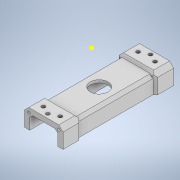
# Autodesk Inventor part: magnet handle top
Saved by Autodesk Inventor 2022 (Build 260153000, 153)
## iProperties
Created: 2022-12-16
Part Number: magnet handle top
Material: Generic
Document SubType Name: Modeling
Designer: chris
Density: 1 g/cm^3
Appearance: Default
Author: chris
Autodesk Inventor part; units mm, degrees
ref_plane "YZ Plane" through (0, 0, 0) normal (1, 0, 0) x (0, 1, 0)
ref_plane "XZ Plane" through (0, 0, 0) normal (0, 1, 0) x (-1, 0, 0)
ref_plane "XY Plane" through (0, 0, 0) normal (0, 0, 1) x (1, 0, 0)
sketch "Sketch1" plane through (0, 0, 0) normal (0, 0, 1) x (1, 0, 0)
  line L0 (0, 0) -> (80, 0)
  line L1 (80, 0) -> (80, 125.359)
  line L2 (60, 200) -> (80, 125.359)
  line L3 (60, 200) -> (137.2741, 200) construction
  line L4 (0, 0) -> (0, 125.359)
  line L5 (20, 200) -> (0, 125.359)
  line L6 (84, 125.8856) -> (84, -4)
  line L7 (84, -4) -> (-4, -4)
  line L8 (-4, -4) -> (-4, 125.8856)
  line L9 (-4, 125.8856) -> (16.9307, 204)
  line L10 (63.0693, 204) -> (84, 125.8856)
  line L11 (20, 204) -> (20, 200)
  line L12 (60, 200) -> (60, 204)
  line L13 (16.9307, 204) -> (20, 204)
  line L14 (60, 204) -> (63.0693, 204)
  point P0 (40, 0)
  dimension "d0" = 80
  dimension "d4" = 75
  dimension "d5" = 4
  constraints: 30 end point, 4 perpendicular, 2 horizontal, 1 equal length, 1 midpoint, 1 vertical, 3 other
  measures "d0" distance of L0.start L0.end
  measures "d4" angle of L2 L3
  measures "d5" distance between parallel lines of L2 L10
extrude "Extrusion1" add sketch "Sketch1" along normal blind 70
sketch "Sketch2" plane through (0, 0, 0) normal (0, 0, -1) x (-1, 0, 0)
  line L0 (-16.9307, 204) -> (4, 125.8856) projected
  line L1 (-84, 125.8856) -> (-63.0693, 204) projected
  line L2 (-16.9307, 204) -> (-63.0693, 204)
  line L3 (-80, 125.359) -> (-80, 0) projected
  line L4 (-60, 200) -> (-80, 125.359) projected
  line L5 (-60, 204) -> (-60, 200) projected
  line L6 (-63.0693, 204) -> (-60, 204) projected
  line L7 (-84, 125.8856) -> (-63.0693, 204) projected
  line L8 (-84, -4) -> (-84, 125.8856) projected
  line L9 (4, -4) -> (-84, -4) projected
  line L10 (4, 125.8856) -> (4, -4) projected
  line L11 (-16.9307, 204) -> (4, 125.8856) projected
  line L12 (-20, 204) -> (-16.9307, 204) projected
  line L13 (-20, 200) -> (-20, 204) projected
  line L14 (0, 125.359) -> (-20, 200) projected
  line L15 (0, 0) -> (0, 125.359) projected
  line L16 (-80, 0) -> (0, 0) projected
  constraints: 2 end point, 1 horizontal
extrude "Extrusion2" add sketch "Sketch2" along normal blind 3
chamfer "Chamfer1" distance 5 angle 45 5 edges at (40, -4, -3) (84, 60.9428, -3) (-4, 60.9428, -3) (6.4653, 164.9428, -3) (73.5347, 164.9428, -3)
chamfer "Chamfer2" distance 3 angle 45 7 edges at (20, 202, 0) (10, 162.6795, 0) (60, 202, 0) (70, 162.6795, 0) (80, 62.6795, 0) (0, 62.6795, 0) (40, 0, 0)
chamfer "Chamfer3" distance 3 angle 45 4 edges at (84, -4, 36) (-4, -4, 36) (0, 0, 36.5) (80, 0, 36.5)
sketch "Sketch3" plane through (0, 0, 70) normal (0, 0, 1) x (1, 0, 0)
  line L0 (77, 0) -> (78.5, 1.5) projected
  line L1 (81, -4) -> (82.5, -2.5) projected
  line L2 (78.5, 1.5) -> (82.5, -2.5)
  line L3 (79, 1) -> (82.5, -2.5) projected
  circle A0 centre (80.75, -0.75) radius 1
  line L4 (-4, -1) -> (-2.5, -2.5) projected
  line L5 (-2.5, -2.5) -> (1.5, 1.5)
  line L6 (0, 3) -> (3, 0) projected
  line L7 (1, 1) -> (-2.5, -2.5) projected
  circle A1 centre (-0.75, -0.75) radius 1
  line L8 (3, 124.964) -> (0, 125.359) projected
  line L9 (16.9307, 204) -> (-4, 125.8856) projected
  line L10 (80, 125.359) -> (77, 124.964) projected
  line L11 (84, -1) -> (84, 125.8856) projected
  line L12 (1, 125.2273) -> (-4, 125.8856) projected
  circle A2 centre (82, 125.6223) radius 1
  circle A3 centre (-2, 125.6223) radius 1
  point P0 (0, 0)
  dimension "d19" = 2
  dimension "d20" = 2
  dimension "d22" = 2
  dimension "d23" = 2
  constraints: 4 centre point, 4 end point, 3 midpoint, 1 perpendicular, 1 point on line
  measures "d19" diameter of A0
  measures "d20" diameter of A1
  measures "d22" diameter of A2
  measures "d23" diameter of A3
extrude "Extrusion3" cut sketch "Sketch3" against normal blind 5
sketch "Sketch4" plane through (22.1071, 204, -3) normal (0, 1, 0) x (1, 0, 0)
  line L0 (35.7859, 0) -> (40.9622, -5) projected
  line L1 (38.374, -2.5) -> (36.3929, -4.5)
  line L2 (34.8929, -3) -> (37.8929, -6) projected
  circle A0 centre (37.3835, -3.5) radius 1
  line L3 (-21.1071, 0) -> (56.8929, 0) projected
  line L4 (17.8929, 0) -> (17.8929, -26)
  circle A1 centre (-1.5976, -3.5) radius 1
  point P0 (-22.1071, -3)
  dimension "d26" = 2
  constraints: 4 end point, 4 midpoint, 2 centre point, 1 symmetric about line, 1 vertical, 1 other
  measures "d26" diameter of A0
extrude "Extrusion4" cut sketch "Sketch4" against normal blind 15
sketch "Sketch5" plane through (0, 0, 0) normal (0, 0, 1) x (1, 0, 0)
  line L0 (77, 3) -> (3, 3) projected
  line L1 (40, 3) -> (40, 43)
  line L2 (40, 43) -> (40, 113)
  line L3 (40, 78) -> (20, 78)
  line L4 (20, 78) -> (20, 55.5)
  line L5 (20, 55.5) -> (60, 55.5)
  line L6 (60, 55.5) -> (60, 100.5)
  line L7 (60, 100.5) -> (20, 100.5)
  line L8 (20, 100.5) -> (20, 78)
  line L9 (40, 78) -> (70, 78)
  line L10 (70, 78) -> (70, 98)
  circle A0 centre (70, 98) radius 1
  line L11 (70, 78) -> (70, 58)
  circle A1 centre (70, 58) radius 1
  circle A2 centre (10, 98) radius 1
  circle A3 centre (10, 58) radius 1
  line L12 (40, 113) -> (40, 133)
  line L13 (40, 133) -> (63.1521, 133)
  line L14 (63.1521, 133) -> (63.1521, 155.7076)
  circle A4 centre (63.1521, 155.7076) radius 1.5
  circle A5 centre (63.1521, 133) radius 1.5
  circle A6 centre (16.8479, 155.7076) radius 1.5
  circle A7 centre (16.8479, 133) radius 1.5
  point P0 (0, 0)
  dimension "d29" = 40
  dimension "d30" = 70
  dimension "d31" = 20
  dimension "d32" = 22.5
  dimension "d33" = 40
  dimension "d34" = 45
  dimension "d35" = 30
  dimension "d36" = 20
  dimension "d37" = 2
  dimension "d38" = 20
  dimension "d39" = 2
  dimension "d40" = 20
  dimension "d41" = 23.1521
  dimension "d42" = 22.7076
  dimension "d43" = 3
  dimension "d44" = 3
  constraints: 28 end point, 8 centre point, 5 perpendicular, 5 vertical, 4 coincident, 4 symmetric about line, 3 horizontal, 2 midpoint, 1 point on line, 4 other
  measures "d29" distance of L1.start L1.end
  measures "d30" distance of L1.end L2.end
  measures "d31" distance of L3.start L3.end
  measures "d32" distance of L3.end L4.end
  measures "d33" distance of L4.end L5.end
  measures "d34" distance of L5.end L6.end
  measures "d35" distance of L3.start L9.end
  measures "d36" distance of L9.end L10.end
  measures "d37" diameter of A0
  measures "d38" distance of L9.end L11.end
  measures "d39" diameter of A1
  measures "d40" distance of L2.end L12.end
  measures "d41" distance of L12.end L13.end
  measures "d42" distance of L13.end L14.end
  measures "d43" diameter of A4
  measures "d44" diameter of A5
extrude "Extrusion5" cut sketch "Sketch5" against normal blind 40
sketch "Sketch7" plane through (-1, -4, 2) normal (0, -1, 0) x (1, 0, 0)
  line L0 (78, 68) -> (4, 68) projected
  line L1 (41, 68) -> (41, 34)
  line L2 (54.7, 34) -> (27.3, 34)
  line L3 (54.7, 34) -> (54.7, 20.8)
  line L4 (54.7, 20.8) -> (27.3, 20.8)
  line L5 (27.3, 34) -> (27.3, 20.8)
  point P0 (1, -2)
  dimension "d47" = 27.4
  dimension "d48" = 34
  dimension "d49" = 13.2
  constraints: 10 end point, 3 vertical, 2 midpoint, 1 coincident, 1 horizontal, 1 horizontal alignment
  measures "d47" distance of L2.start L2.end
  measures "d48" distance of L1.start L1.end
  measures "d49" distance of L2.start L3.end
extrude "Extrusion6" cut sketch "Sketch7" against normal blind 27.4
sketch "Sketch8" plane through (-4, 125.8856, 2) normal (-0.9659258, 0.258819, 0) x (0, 0, 1)
  line L0 (-2, 13.7678) -> (-2, 10.7678) projected
  line L1 (-2, 35.7017) -> (-2, 32.7017) projected
  line L2 (3.9828, 34.5121) -> (3.9828, 12.5782)
  line L3 (3.9828, 23.5451) -> (5.9828, 23.5451)
  line L4 (5.9828, 23.5451) -> (12.9828, 23.5451)
  line L5 (12.9828, 23.5451) -> (12.9828, 30.2951)
  line L6 (12.9828, 30.2951) -> (12.9828, 16.7951)
  line L7 (12.9828, 16.7951) -> (5.9828, 16.7951)
  line L8 (5.9828, 16.7951) -> (5.9828, 29.9848)
  line L9 (5.9828, 29.9848) -> (12.9828, 30.2951)
  point P0 (-2, -120.5609)
  point P1 (12.9828, 30.2951)
  dimension "d52" = 2
  dimension "d53" = 7
  dimension "d54" = 6.75
  dimension "d55" = 13.5
  constraints: 16 end point, 3 perpendicular, 3 point on line, 1 coincident, 1 horizontal, 1 midpoint, 1 vertical
  measures "d52" distance of L3.start L3.end
  measures "d53" distance of L3.end L4.end
  measures "d54" distance of L4.end L5.end
  measures "d55" distance of L5.end L6.end
extrude "Extrusion7" cut sketch "Sketch8" against normal blind 9
chamfer "Chamfer4" distance 1 angle 45 4 edges at (5.7728, 154.6308, 14.9828) (2.2788, 141.5908, 14.9828) (2.2788, 141.5908, 7.9828) (5.6925, 154.331, 7.9828)
sketch "Sketch9" plane through (-4, 125.8856, 2) normal (-1, 0, 0) x (0, 0, 1)
  line L0 (1, -0.5266) -> (1, -122.8856) projected
  line L1 (1, -48.8247) -> (7.6436, -48.8247)
  line L2 (7.6436, -48.8247) -> (7.6436, -34.3247)
  line L3 (7.6436, -34.3247) -> (7.6436, -63.3247)
  circle A0 centre (7.6436, -34.3247) radius 2
  circle A1 centre (7.6436, -63.3247) radius 2
  point P0 (-2, -125.8856)
  dimension "d61" = 14.5
  dimension "d62" = 29
  dimension "d63" = 4
  dimension "d64" = 4
  constraints: 6 end point, 2 centre point, 2 coincident, 2 point on line, 1 horizontal, 1 perpendicular
  measures "d61" distance of L1.end L2.end
  measures "d62" distance of L2.end L3.end
  measures "d63" diameter of A0
  measures "d64" diameter of A1
extrude "Extrusion8" cut sketch "Sketch9" against normal blind 999
sketch "Sketch17" plane through (0, 0, -3) normal (0, 0, -1) x (-1, 0, 0)
  line L0 (-60, 55.5) -> (-60, 100.5) projected
  line L1 (-60, 78) -> (-77, 78)
  line L2 (-77, 124.964) -> (-77, 3) projected
  line L3 (-77, 78) -> (-77, 43)
  line L4 (-77, 78) -> (-77, 113)
  line L5 (-60, 55.5) -> (-20, 55.5) projected
  line L6 (-40, 55.5) -> (-40, 37.7198)
  line L7 (-20, 55.5) -> (-20, 100.5)
  line L8 (-20, 78) -> (-3, 78)
  line L9 (-3, 78) -> (-3, 43)
  line L10 (-3, 78) -> (-3, 113)
  line L11 (-20, 55.5) -> (-60, 55.5)
  line L12 (-77, 43) -> (-3, 43)
  line L13 (-3, 3) -> (-3, 124.964) projected
  line L14 (-3, 113) -> (-77, 113)
  line L15 (-79, 1) -> (-79, 125.2273) projected
  circle A0 centre (-63.1521, 133) radius 1.5 projected
  circle A1 centre (-70, 98) radius 1 projected
  circle A2 centre (-10, 58) radius 1 projected
  circle A3 centre (-16.8479, 133) radius 1.5 projected
  circle A4 centre (-63.1521, 155.7076) radius 1.5 projected
  circle A5 centre (-70, 58) radius 1 projected
  circle A6 centre (-10, 98) radius 1 projected
  circle A7 centre (-16.8479, 155.7076) radius 1.5 projected
  line L16 (-20, 55.5) -> (-60, 55.5) projected
  line L17 (-60, 55.5) -> (-60, 100.5) projected
  line L18 (-60, 100.5) -> (-20, 100.5) projected
  line L19 (-20, 100.5) -> (-20, 55.5) projected
  line L20 (-79, 125.2273) -> (-57.8929, 204) projected
  line L21 (-79, 1) -> (-79, 125.2273) projected
  line L22 (-1, 1) -> (-79, 1) projected
  line L23 (-1, 125.2273) -> (-1, 1) projected
  line L24 (-22.1071, 204) -> (-1, 125.2273) projected
  line L25 (-22.1071, 204) -> (-57.8929, 204) projected
  point P0 (0, 0)
  dimension "d106" = 35
  dimension "d107" = 35
  constraints: 22 end point, 7 symmetric about line, 3 perpendicular, 3 vertical, 2 midpoint, 1 point on line
  measures "d106" distance of L1.end L3.end
  measures "d107" distance of L1.end L4.end
extrude "Extrusion16" add sketch "Sketch17" along normal blind 3 contours L5 L6 L12 L2 L1 L0 | L0 L18 L7 L5 | L1 L2 L14 L10 L8 L7 L18 L0 | L5 L7 L8 L9 L12 L6
sketch "Sketch18" plane through (0, 0, 70) normal (0, 0, 1) x (1, 0, 0)
  line L0 (-145.0841, -156.9657) -> (0, 339.906)
  line L1 (0, 339.906) -> (209.9789, 212.1699)
  line L2 (209.9789, 212.1699) -> (104.9894, -207.8436)
  line L3 (104.9894, -207.8436) -> (-145.0841, -156.9657)
  point P0 (0, 0)
  constraints: 8 end point
extrude "Extrusion17" cut sketch "Sketch18" against normal blind 73
sketch "Sketch19" plane through (0, 0, -3) normal (0, 0, 1) x (1, 0, 0)
  line L0 (3, 113) -> (77, 113) projected
  line L1 (77, 43) -> (3, 43) projected
  line L2 (40, 43) -> (40, 113)
  line L3 (40, 78) -> (25, 78)
  line L4 (25, 78) -> (25, 63)
  line L5 (25, 63) -> (40, 63)
  line L6 (40, 63) -> (55, 63)
  line L7 (55, 63) -> (55, 93)
  line L8 (55, 93) -> (25, 93)
  line L9 (25, 93) -> (25, 78)
  line L10 (22, 78) -> (22, 60)
  line L11 (22, 60) -> (40, 60)
  line L12 (40, 60) -> (58, 60)
  line L13 (58, 60) -> (58, 96)
  line L14 (58, 96) -> (22, 96)
  line L15 (22, 96) -> (22, 78)
  point P0 (0, 0)
  dimension "d112" = 15
  dimension "d113" = 15
  dimension "d114" = 15
  dimension "d115" = 15
  dimension "d116" = 30
  dimension "d117" = 3
  constraints: 28 end point, 6 perpendicular, 3 midpoint, 3 point on line, 1 horizontal, 5 other
  measures "d112" distance of L3.start L3.end
  measures "d113" distance of L3.end L4.end
  measures "d114" distance of L4.end L5.end
  measures "d115" distance of L5.end L6.end
  measures "d116" distance of L6.end L7.end
  measures "d117" distance between parallel lines of L9 L15
extrude "Extrusion18" add sketch "Sketch19" along normal blind 73 contours L11 L10 L15 L14 L2 L8 L9 L4 L5 | L2 L6 L7 L8 L14 L13 L12
sketch "Sketch20" plane through (0, 0, -3) normal (0, 0, 1) x (1, 0, 0)
  line L0 (25, 93) -> (25, 63) projected
  line L1 (25, 63) -> (55, 63) projected
  line L2 (55, 63) -> (55, 93) projected
  line L3 (55, 93) -> (25, 93) projected
  point P0 (0, 0)
extrude "Extrusion19" cut sketch "Sketch20" against normal blind 73
chamfer "Chamfer7" distance 3 angle 45 8 edges at (58, 60, 33.5) (25, 93, 32) (58, 96, 33.5) (55, 63, 32) (22, 96, 33.5) (55, 93, 32) (25, 63, 32) (22, 60, 33.5)
chamfer "Chamfer8" distance 3 angle 45 4 edges at (3, 78, -3) (40, 43, -3) (77, 78, -3) (40, 113, -3)
sketch "Sketch21" plane through (25, 96, -3) normal (0, 1, 0) x (1, 0, 0)
  line L0 (0, -73) -> (0, 0) projected
  line L1 (30, -73) -> (0, -73) projected
  line L2 (30, 0) -> (30, -73) projected
  line L3 (0, 0) -> (30, 0) projected
  line L4 (0, -73) -> (0, 3) projected
  line L5 (0, -35) -> (30, -35)
  line L6 (30, -73) -> (30, 0) projected
  circle A0 centre (15, -35) radius 9.425
  point P0 (-25, -3)
  dimension "d128" = 18.85
  constraints: 2 end point, 2 midpoint, 1 centre point, 1 perpendicular, 1 point on line
  measures "d128" diameter of A0
extrude "Extrusion20" cut sketch "Sketch21" against normal blind 3 contours A0 L5 | L5 A0
sketch "Sketch22" plane through (0, 0, 70) normal (0, 0, 1) x (1, 0, 0)
  line L0 (25, 60) -> (22, 63) projected
  line L1 (25, 60) -> (55, 60) projected
  line L2 (58, 63) -> (55, 60) projected
  line L3 (58, 63) -> (58, 93) projected
  line L4 (55, 96) -> (58, 93) projected
  line L5 (55, 96) -> (25, 96) projected
  line L6 (22, 93) -> (25, 96) projected
  line L7 (22, 93) -> (22, 63) projected
  line L8 (28, 93) -> (52, 93) projected
  line L9 (55, 90) -> (52, 93) projected
  line L10 (55, 90) -> (55, 66) projected
  line L11 (52, 63) -> (55, 66) projected
  line L12 (52, 63) -> (28, 63) projected
  line L13 (25, 66) -> (28, 63) projected
  line L14 (25, 66) -> (25, 90) projected
  line L15 (28, 93) -> (25, 90) projected
  line L16 (25, 90) -> (28, 93) projected
  line L17 (26.5, 91.5) -> (23.5, 94.5)
  line L18 (22, 93) -> (25, 96) projected
  line L19 (25, 60) -> (22, 63) projected
  line L20 (23.5, 61.5) -> (26.5, 64.5)
  line L21 (28, 63) -> (25, 66) projected
  line L22 (56.5, 61.5) -> (53.5, 64.5)
  line L23 (53.5, 91.5) -> (56.5, 94.5)
  line L24 (58, 93) -> (55, 96) projected
  circle A0 centre (25, 63) radius 1
  circle A1 centre (55, 63) radius 1
  circle A2 centre (55, 93) radius 1
  circle A3 centre (25, 93) radius 1
  point P0 (0, 0)
  dimension "d131" = 2
  dimension "d132" = 2
  dimension "d133" = 2
  dimension "d134" = 2
  constraints: 12 midpoint, 8 end point, 4 centre point, 1 point on line
  measures "d131" diameter of A0
  measures "d132" diameter of A1
  measures "d133" diameter of A2
  measures "d134" diameter of A3
extrude "Extrusion21" cut sketch "Sketch22" against normal blind 200 contours A0 L20 | L20 A0 | A1 L22 | L22 A1 | A3 L17 | L17 A3 | A2 L23 | L23 A2
sketch "Sketch23" plane through (0, 0, -3) normal (0, 0, 1) x (1, 0, 0)
  line L0 (25, 96) -> (55, 96) projected
  line L1 (58, 93) -> (55, 96) projected
  line L2 (58, 93) -> (58, 63) projected
  line L3 (55, 60) -> (58, 63) projected
  line L4 (55, 60) -> (25, 60) projected
  line L5 (22, 63) -> (25, 60) projected
  line L6 (22, 63) -> (22, 93) projected
  line L7 (25, 96) -> (22, 93) projected
  circle A0 centre (10, 98) radius 1 projected
  circle A1 centre (70, 58) radius 1 projected
  circle A2 centre (10, 58) radius 1 projected
  circle A3 centre (70, 98) radius 1 projected
  line L8 (6, 110) -> (74, 110) projected
  line L9 (6, 46) -> (6, 110) projected
  line L10 (74, 46) -> (6, 46) projected
  line L11 (74, 110) -> (74, 46) projected
  line L12 (6, 46) -> (6, 110) projected
  line L13 (3, 113) -> (6, 110) projected
  line L14 (3, 43) -> (3, 113) projected
  line L15 (6, 46) -> (3, 43) projected
  line L16 (74, 46) -> (6, 46) projected
  line L17 (6, 46) -> (3, 43) projected
  line L18 (77, 43) -> (3, 43) projected
  line L19 (77, 43) -> (74, 46) projected
  line L20 (3, 113) -> (77, 113) projected
  line L21 (3, 113) -> (6, 110) projected
  line L22 (6, 110) -> (74, 110) projected
  line L23 (77, 113) -> (74, 110) projected
  line L24 (74, 110) -> (74, 46) projected
  line L25 (77, 43) -> (74, 46) projected
  line L26 (77, 113) -> (77, 43) projected
  line L27 (77, 113) -> (74, 110) projected
  point P0 (0, 0)
extrude "Extrusion22" cut sketch "Sketch23" against normal blind 10
sketch "Sketch25" plane through (25, 96, 70) normal (0, 1, 0) x (1, 0, 0)
  point P0 (-25, 70)
sketch "Sketch24" plane through (0, 0, -6) normal (0, 0, -1) x (-1, 0, 0)
  line L0 (-22, 93) -> (-25, 96) projected
  line L1 (-25, 96) -> (-55, 96) projected
  line L2 (-55, 96) -> (-58, 93) projected
  line L3 (-58, 93) -> (-58, 63) projected
  line L4 (-58, 63) -> (-55, 60) projected
  line L5 (-55, 60) -> (-25, 60) projected
  line L6 (-25, 60) -> (-22, 63) projected
  line L7 (-22, 63) -> (-22, 93) projected
  circle A0 centre (-25, 93) radius 1 projected
  circle A1 centre (-25, 63) radius 1 projected
  circle A2 centre (-55, 93) radius 1 projected
  circle A3 centre (-55, 63) radius 1 projected
  line L8 (-55, 66) -> (-55, 90) projected
  line L9 (-52, 93) -> (-55, 90) projected
  line L10 (-52, 93) -> (-28, 93) projected
  line L11 (-25, 90) -> (-28, 93) projected
  line L12 (-25, 90) -> (-25, 66) projected
  line L13 (-28, 63) -> (-25, 66) projected
  line L14 (-28, 63) -> (-52, 63) projected
  line L15 (-55, 66) -> (-52, 63) projected
  point P0 (0, 0)
extrude "Extrusion23" add sketch "Sketch24" along normal blind 20.75
sketch "Sketch26" plane through (0, 0, 70) normal (0, 0, 1) x (1, 0, 0)
  circle A0 centre (25, 93) radius 1 projected
  circle A1 centre (25, 63) radius 1 projected
  circle A2 centre (55, 93) radius 1 projected
  circle A3 centre (55, 63) radius 1 projected
  line L0 (25, 60) -> (22, 63) projected
  line L1 (25, 60) -> (55, 60) projected
  line L2 (58, 63) -> (55, 60) projected
  line L3 (58, 63) -> (58, 93) projected
  line L4 (55, 96) -> (58, 93) projected
  line L5 (55, 96) -> (25, 96) projected
  line L6 (22, 93) -> (25, 96) projected
  line L7 (22, 93) -> (22, 63) projected
  line L8 (28, 93) -> (52, 93) projected
  line L9 (55, 90) -> (52, 93) projected
  line L10 (55, 90) -> (55, 66) projected
  line L11 (52, 63) -> (55, 66) projected
  line L12 (52, 63) -> (28, 63) projected
  line L13 (25, 66) -> (28, 63) projected
  line L14 (25, 66) -> (25, 90) projected
  line L15 (28, 93) -> (25, 90) projected
  point P0 (0, 0)
extrude "Extrusion24" add sketch "Sketch26" along normal blind 20.75
sketch "Sketch28" plane through (25, 96, -26.75) normal (0, 1, 0) x (1, 0, 0)
  point P0 (-25, -26.75)
sketch "Sketch37" plane through (0, 0, -26.75) normal (0, 0, -1) x (-1, 0, 0)
  line L0 (-25, 96) -> (-55, 96) projected
  line L1 (-55, 96) -> (-58, 93) projected
  line L2 (-58, 93) -> (-58, 63) projected
  line L3 (-58, 63) -> (-55, 60) projected
  line L4 (-55, 60) -> (-25, 60) projected
  line L5 (-25, 60) -> (-22, 63) projected
  line L6 (-22, 63) -> (-22, 93) projected
  line L7 (-22, 93) -> (-25, 96) projected
  line L8 (-28, 63) -> (-52, 63) projected
  line L9 (-52, 63) -> (-55, 66) projected
  line L10 (-55, 66) -> (-55, 90) projected
  line L11 (-55, 90) -> (-52, 93) projected
  line L12 (-52, 93) -> (-28, 93) projected
  line L13 (-28, 93) -> (-25, 90) projected
  line L14 (-25, 90) -> (-25, 66) projected
  line L15 (-25, 66) -> (-28, 63) projected
  circle A0 centre (-55, 63) radius 1 projected
  circle A1 centre (-55, 93) radius 1 projected
  circle A2 centre (-25, 63) radius 1 projected
  circle A3 centre (-25, 93) radius 1 projected
  point P0 (0, 0)
extrude "Extrusion27" add sketch "Sketch37" along normal blind 0.25
sketch "Sketch38" plane through (0, 0, 90.75) normal (0, 0, 1) x (1, 0, 0)
  line L0 (58, 93) -> (55, 96) projected
  line L1 (55, 96) -> (25, 96) projected
  line L2 (25, 96) -> (22, 93) projected
  line L3 (22, 93) -> (22, 63) projected
  line L4 (22, 63) -> (25, 60) projected
  line L5 (25, 60) -> (55, 60) projected
  line L6 (55, 60) -> (58, 63) projected
  line L7 (58, 63) -> (58, 93) projected
  line L8 (25, 66) -> (25, 90) projected
  line L9 (25, 90) -> (28, 93) projected
  line L10 (28, 93) -> (52, 93) projected
  line L11 (52, 93) -> (55, 90) projected
  line L12 (55, 90) -> (55, 66) projected
  line L13 (55, 66) -> (52, 63) projected
  line L14 (52, 63) -> (28, 63) projected
  line L15 (28, 63) -> (25, 66) projected
  circle A0 centre (55, 63) radius 1 projected
  circle A1 centre (55, 93) radius 1 projected
  circle A2 centre (25, 63) radius 1 projected
  circle A3 centre (25, 93) radius 1 projected
  point P0 (0, 0)
extrude "Extrusion28" add sketch "Sketch38" along normal blind 0.25
sketch "Sketch40" plane through (0, 0, 91) normal (0, 0, 1) x (1, 0, 0)
  line L0 (55, 96) -> (25, 96) projected
  line L1 (25, 96) -> (22, 93) projected
  line L2 (22, 93) -> (22, 63) projected
  line L3 (22, 63) -> (25, 60) projected
  line L4 (25, 60) -> (55, 60) projected
  line L5 (55, 60) -> (58, 63) projected
  line L6 (58, 63) -> (58, 93) projected
  line L7 (58, 93) -> (55, 96) projected
  circle A0 centre (25, 93) radius 1 projected
  circle A1 centre (25, 63) radius 1 projected
  circle A2 centre (55, 93) radius 1 projected
  circle A3 centre (55, 63) radius 1 projected
  line L8 (25, 66) -> (25, 90) projected
  line L9 (25, 90) -> (28, 93) projected
  line L10 (28, 93) -> (52, 93) projected
  line L11 (52, 93) -> (55, 90) projected
  line L12 (55, 90) -> (55, 66) projected
  line L13 (55, 66) -> (52, 63) projected
  line L14 (52, 63) -> (28, 63) projected
  line L15 (28, 63) -> (25, 66) projected
  point P0 (0, 0)
extrude "Extrusion29" add sketch "Sketch40" against normal up to surface (118 mm away) contours A0 | A1 | A2 | A3
sketch "Sketch42" plane through (0, 0, 91) normal (0, 0, 1) x (1, 0, 0)
  line L0 (55, 96) -> (25, 96) projected
  line L1 (25, 96) -> (22, 93) projected
  line L2 (22, 93) -> (22, 63) projected
  line L3 (22, 63) -> (25, 60) projected
  line L4 (25, 60) -> (55, 60) projected
  line L5 (55, 60) -> (58, 63) projected
  line L6 (58, 63) -> (58, 93) projected
  line L7 (58, 93) -> (55, 96) projected
  line L8 (25, 66) -> (25, 90) projected
  line L9 (25, 90) -> (28, 93) projected
  line L10 (28, 93) -> (52, 93) projected
  line L11 (52, 93) -> (55, 90) projected
  line L12 (55, 90) -> (55, 66) projected
  line L13 (55, 66) -> (52, 63) projected
  line L14 (52, 63) -> (28, 63) projected
  line L15 (28, 63) -> (25, 66) projected
  line L16 (23.9645, 98.5) -> (56.0355, 98.5)
  line L17 (56.0355, 98.5) -> (60.5, 94.0355)
  line L18 (60.5, 94.0355) -> (60.5, 61.9645)
  line L19 (60.5, 61.9645) -> (56.0355, 57.5)
  line L20 (56.0355, 57.5) -> (23.9645, 57.5)
  line L21 (23.9645, 57.5) -> (19.5, 61.9645)
  line L22 (19.5, 61.9645) -> (19.5, 94.0355)
  line L23 (19.5, 94.0355) -> (23.9645, 98.5)
  point P0 (0, 0)
  dimension "d153" = 2.5
  constraints: 16 end point, 7 other
  measures "d153" distance between parallel lines of L0 L16
extrude "Extrusion30" add sketch "Sketch42" against normal blind 20 contours L16 L17 L18 L19 L20 L21 L22 L23
sketch "Sketch43" plane through (0, 0, -27) normal (0, 0, -1) x (-1, 0, 0)
  line L0 (-55, 96) -> (-58, 93) projected
  line L1 (-58, 93) -> (-58, 63) projected
  line L2 (-58, 63) -> (-55, 60) projected
  line L3 (-55, 60) -> (-25, 60) projected
  line L4 (-25, 60) -> (-22, 63) projected
  line L5 (-22, 63) -> (-22, 93) projected
  line L6 (-22, 93) -> (-25, 96) projected
  line L7 (-25, 96) -> (-55, 96) projected
  line L8 (-28, 63) -> (-52, 63) projected
  line L9 (-52, 63) -> (-55, 66) projected
  line L10 (-55, 66) -> (-55, 90) projected
  line L11 (-55, 90) -> (-52, 93) projected
  line L12 (-52, 93) -> (-28, 93) projected
  line L13 (-28, 93) -> (-25, 90) projected
  line L14 (-25, 90) -> (-25, 66) projected
  line L15 (-25, 66) -> (-28, 63) projected
  line L16 (-56.0355, 98.5) -> (-60.5, 94.0355)
  line L17 (-60.5, 94.0355) -> (-60.5, 61.9645)
  line L18 (-60.5, 61.9645) -> (-56.0355, 57.5)
  line L19 (-56.0355, 57.5) -> (-23.9645, 57.5)
  line L20 (-23.9645, 57.5) -> (-19.5, 61.9645)
  line L21 (-19.5, 61.9645) -> (-19.5, 94.0355)
  line L22 (-19.5, 94.0355) -> (-23.9645, 98.5)
  line L23 (-23.9645, 98.5) -> (-56.0355, 98.5)
  point P0 (0, 0)
  dimension "d156" = 2.5
  constraints: 16 end point, 7 other
  measures "d156" distance between parallel lines of L7 L23
extrude "Extrusion31" add sketch "Sketch43" against normal blind 20 contours L23 L22 L21 L20 L19 L18 L17 L16
chamfer "Chamfer9" distance 3 angle 45 8 edges at (40, 57.5, -7) (60.5, 78, -7) (60.5, 78, 71) (40, 98.5, -7) (40, 98.5, 71) (19.5, 78, 71) (19.5, 78, -7) (40, 57.5, 71)
sketch "Sketch46" plane through (0, 0, -27) normal (0, 0, -1) x (-1, 0, 0)
  line L0 (-23.9645, 57.5) -> (-19.5, 61.9645) projected
  line L1 (-21.7322, 59.7322) -> (-26.5, 64.5)
  line L2 (-25, 66) -> (-28, 63) projected
  circle A0 centre (-24.1161, 62.1161) radius 1.5
  line L3 (-30.575, 93) -> (-49.425, 93) projected
  line L4 (-28, 63) -> (-52, 63) projected
  circle A1 centre (-24.1161, 93.8839) radius 1.5
  circle A2 centre (-55.8839, 93.8839) radius 1.5
  circle A3 centre (-55.8839, 62.1161) radius 1.5
  point P0 (0, 0)
  point P1 (-40, 78)
  dimension "d162" = 3
  dimension "d165" = 360
  constraints: 4 centre point, 3 midpoint, 2 end point, 9 other
  measures "d162" diameter of A0
extrude "Extrusion32" cut sketch "Sketch46" against normal blind 15
sketch "Sketch48" plane through (0, 0, 91) normal (0, 0, 1) x (1, 0, 0)
  line L0 (56.0355, 57.5) -> (60.5, 61.9645)
  line L1 (58.2678, 59.7322) -> (53.5, 64.5)
  line L2 (55, 66) -> (52, 63)
  circle A0 centre (55.8839, 62.1161) radius 1.5
  line L3 (-30.575, 93) -> (-49.425, 93)
  line L4 (52, 63) -> (28, 63)
  circle A1 centre (55.8839, 93.8839) radius 1.5
  circle A2 centre (24.1161, 93.8839) radius 1.5
  circle A3 centre (24.1161, 62.1161) radius 1.5
  line L5 (55, 90) -> (55, 66) projected
  line L6 (28, 93) -> (52, 93) projected
  point P0 (0, 0)
  point P1 (40, 78)
  point P2 (55, 78)
  point P3 (40, 93)
  dimension "d171" = 3
  dimension "d172" = 360
  constraints: 10 end point, 5 midpoint, 4 centre point, 1 horizontal alignment, 1 vertical alignment, 9 other
  measures "d171" diameter of A0
extrude "Extrusion33" cut sketch "Sketch48" against normal blind 15
sketch "Sketch49" plane through (23.9645, 57.5, 91) normal (0, -1, 0) x (1, 0, 0)
  line L0 (0, 0) -> (32.0711, 0) projected
  line L1 (32.0711, -17) -> (0, -17) projected
  line L2 (16.0355, -8.5) -> (25.0355, -8.5)
  line L3 (28.0355, -118) -> (28.0355, 0) projected
  circle A0 centre (25.0355, -8.5) radius 2
  circle A1 centre (7.0355, -8.5) radius 2
  line L4 (28.0355, -59) -> (79.5014, -59)
  line L5 (16.0355, -8.5) -> (16.0355, 0)
  circle A2 centre (16.0355, -4.25) radius 2
  line L6 (16.0355, -109.5) -> (25.0355, -109.5)
  line L7 (28.0355, 0) -> (28.0355, -118)
  circle A3 centre (25.0355, -109.5) radius 2
  circle A4 centre (7.0355, -109.5) radius 2
  line L8 (16.0355, -109.5) -> (16.0355, -118)
  circle A5 centre (16.0355, -113.75) radius 2
  point P0 (-23.9645, -91)
  dimension "d175" = 9
  dimension "d176" = 4
  dimension "d177" = 4
  constraints: 12 end point, 8 symmetric about line, 6 centre point, 3 midpoint, 2 coincident, 1 horizontal, 1 perpendicular, 3 other
  measures "d175" distance of L2.start L2.end
  measures "d176" diameter of A0
  measures "d177" diameter of A2
extrude "Extrusion34" cut sketch "Sketch49" against normal through all
sketch "Sketch50" plane through (60.5, 61.9645, 91) normal (1, 0, 0) x (0, 0, -1)
  line L0 (0, 28.0355) -> (0, 4.0355) projected
  line L1 (0, 16.0355) -> (-51.4924, 1.0144)
  line L2 (-51.4924, 1.0144) -> (-29.6043, -61.9645)
  line L3 (-29.6043, -61.9645) -> (173.5524, -23.1845)
  line L4 (173.5524, -23.1845) -> (159.9216, 16.0355)
  line L5 (159.9216, 16.0355) -> (118, 16.0355)
  line L6 (118, 28.0355) -> (118, 4.0355) projected
  line L7 (118, 16.0355) -> (0, 16.0355)
  point P0 (91, -61.9645)
  constraints: 12 end point, 2 midpoint, 1 collinear, 1 parallel
extrude "Extrusion35" cut sketch "Sketch50" against normal through all
equation "\"d45\" = d33"
equation "\"d50\" = d47"
body "Solid1"
